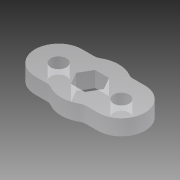
# Autodesk Inventor part: plastic_part_99
Saved by Autodesk Inventor 2013 (Build 170138000, 138)
## iProperties
Shininess: 20.0
Created: 2013-06-02
Part Number: plastic_part_99
Document SubType Name: Modeling
Designer: Noa Izumi
Material: Default
Density: 1 g/cm^3
Density: 0.0
Volumn: 0.0
Area: 0.0
PropertySet Name: Model Information
Control State: 0
Master: False
Checked Out: False
Author: Noa Izumi
Autodesk Inventor part; units mm, degrees
ref_plane "YZ Plane" through (0, 0, 0) normal (1, 0, 0) x (0, 1, 0)
ref_plane "XZ Plane" through (0, 0, 0) normal (0, 1, 0) x (-1, 0, 0)
ref_plane "XY Plane" through (0, 0, 0) normal (0, 0, 1) x (1, 0, 0)
sketch "Sketch1" plane through (0, 0, 0) normal (0, 0, 1) x (1, 0, 0)
  circle A0 centre (0, 0) radius 5.5
  arc A1 (6, -4.5) -> (6, 4.5) centre (6, 0) ccw
  arc A2 (-6, 4.5) -> (-6, -4.5) centre (-6, 0) ccw
  line L0 (-6, 4.5) -> (6, 4.5)
  line L1 (6, -4.5) -> (-6, -4.5)
  dimension "d0" = 11
  dimension "d5" = 9
  dimension "d6" = 6
  dimension "d7" = 9
  dimension "d8" = 6
  constraints: 4 end point, 4 point on circle, 3 centre point, 1 horizontal, 1 parallel
  measures "d0" diameter of A0
  measures "d5" diameter of A1
  measures "d6" distance of A1.centre A0.centre
  measures "d7" diameter of A2
  measures "d8" distance of A0.centre A2.centre
extrude "Extrusion1" add sketch "Sketch1" along normal blind 3
fillet "圓角1" radius 2 4 edges at (3.1623, -4.5, 1.5) (-3.1623, -4.5, 1.5) (3.1623, 4.5, 1.5) (-3.1623, 4.5, 1.5)
sketch "草圖3" plane through (0, 0, 3) normal (0, 0, 1) x (1, 0, 0)
  arc A0 (-6, 4.5) -> (-6, -4.5) centre (-6, 0) ccw projected
  arc A1 (6, -4.5) -> (6, 4.5) centre (6, 0) ccw projected
  constraints: 2 coincident
hole "孔1" at (-6, 0, 3) at (6, 0, 3) direction (0, 0, -1) diameter 3 end through all
sketch "草圖4" plane through (0, 0, 3) normal (0, 0, 1) x (1, 0, 0)
  arc A0 (2.7439, 4.7667) -> (-2.7439, 4.7667) centre (0, 0) ccw projected
  line L0 (1.3279, 2.3) -> (2.6558, 0)
  line L1 (2.6558, 0) -> (1.3279, -2.3)
  line L2 (1.3279, -2.3) -> (-1.3279, -2.3)
  line L3 (-1.3279, -2.3) -> (-2.6558, 0)
  line L4 (-2.6558, 0) -> (-1.3279, 2.3)
  line L5 (-1.3279, 2.3) -> (1.3279, 2.3)
  dimension "d17" = 4.6
  constraints: 12 end point, 1 coincident, 13 other
  measures "d17" distance between parallel lines of L2 L5
extrude "擠出2" cut sketch "草圖4" against normal through all
